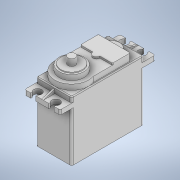
# Autodesk Inventor part: HS-485HB
Saved by Autodesk Inventor 2020 (Build 240168000, 168)
## iProperties
Created: 2023-02-03
Part Number: HS-485HB
Material: Generic
Document SubType Name: Modeling
Designer: legoo
Density: 1 g/cm^3
Appearance: Default
Author: legoo
Autodesk Inventor part; units mm, degrees
ref_plane "YZ Plane" through (0, 0, 0) normal (1, 0, 0) x (0, 1, 0)
ref_plane "XZ Plane" through (0, 0, 0) normal (0, 1, 0) x (-1, 0, 0)
sketch "Sketch1" plane through (0, 0, 0) normal (0, 1, 0) x (-1, 0, 0)
  line L0 (0, 0) -> (19.8, 0)
  line L1 (19.8, 0) -> (19.8, -40.2)
  line L2 (19.8, -40.2) -> (0, -40.2)
  line L3 (0, -40.2) -> (0, 0)
  dimension "d0" = 40.2
  dimension "d1" = 19.8
  constraints: 8 end point, 2 parallel, 1 horizontal, 1 perpendicular
  measures "d0" distance of L2.end L0.start
  measures "d1" distance of L0.start L0.end
extrude "Extrusion1" add sketch "Sketch1" along normal blind 27.7
sketch "Sketch2" plane through (0, 27.7, 0) normal (0, 1, 0) x (1, 0, 0)
  line L0 (-19.8, -6.4) -> (0, -6.4)
  line L1 (0, -6.4) -> (0, 46.6)
  line L2 (0, 46.6) -> (-19.8, 46.6)
  line L3 (-19.8, 46.6) -> (-19.8, -6.4)
  line L4 (-19.8, 40.2) -> (-19.8, 0) projected
  line L5 (0, 0) -> (0, 40.2) projected
  line L6 (-19.8, 0) -> (0, 0) projected
  dimension "d4" = 0
  dimension "d5" = 0
  dimension "d6" = 53
  dimension "d7" = 6.4
  constraints: 8 end point, 2 parallel, 1 horizontal, 1 perpendicular
  measures "d4" distance between parallel lines of L3 L4
  measures "d5" distance between parallel lines of L1 L5
  measures "d6" distance between parallel lines of L0 L2
  measures "d7" distance between parallel lines of L0 L6
extrude "Extrusion2" add sketch "Sketch2" along normal blind 2.6
sketch "Sketch3" plane through (0, 30.3, 0) normal (0, 1, 0) x (1, 0, 0)
  arc A0 (-13.5375, -5.6705) -> (-16.4375, -5.6705) centre (-14.9875, -3.95) ccw
  arc A1 (-3.4, -5.6705) -> (-6.3, -5.6705) centre (-4.85, -3.95) ccw
  arc A2 (-16.4, 45.8705) -> (-13.5, 45.8705) centre (-14.95, 44.15) ccw
  arc A3 (-6.3, 45.8705) -> (-3.4, 45.8705) centre (-4.85, 44.15) ccw
  line L0 (0, -6.4) -> (0, 46.6) projected
  line L1 (0, 46.6) -> (-19.8, 46.6) projected
  line L2 (-16.4375, -5.6705) -> (-16.4375, -6.4)
  line L3 (-13.5375, -5.6705) -> (-13.5375, -6.4)
  line L4 (-19.8, -6.4) -> (0, -6.4) projected
  line L5 (-16.4375, -6.4) -> (-13.5375, -6.4)
  line L6 (-6.3, -5.6705) -> (-6.3, -6.4)
  line L7 (-3.4, -5.6705) -> (-3.4, -6.4)
  line L8 (-6.3, -6.4) -> (-3.4, -6.4)
  line L9 (-16.4, 46.6) -> (-16.4, 45.8705)
  line L10 (-13.5, 45.8705) -> (-13.5, 46.6)
  line L11 (-6.3, 45.8705) -> (-6.3, 46.6)
  line L12 (-3.4, 45.8705) -> (-3.4, 46.6)
  line L13 (-16.4, 46.6) -> (-13.5, 46.6)
  line L14 (-6.3, 46.6) -> (-3.4, 46.6)
  point P0 (0, 0)
  dimension "d10" = 4.5
  dimension "d11" = 48.1
  dimension "d12" = 48.1
  dimension "d13" = 10.1
  dimension "d14" = 4.85
  dimension "d15" = 4.85
  dimension "d16" = 2.45
  dimension "d17" = 2.45
  dimension "d18" = 2.9
  dimension "d19" = 1.45
  dimension "d20" = 2.9
  dimension "d21" = 1.45
  dimension "d22" = 2.9
  dimension "d23" = 2.9
  dimension "d24" = 1.45
  dimension "d25" = 1.45
  constraints: 24 end point, 8 point on circle, 8 point on line, 7 vertical, 4 centre point, 3 equal radius, 1 perpendicular
  measures "d10" diameter of A0
  measures "d11" distance of A3.centre A1.centre
  measures "d12" distance of A0.centre A2.centre
  measures "d13" distance of A3.centre A2.centre
  measures "d14" distance from line of L0 A1.centre
  measures "d15" distance from line of L0 A3.centre
  measures "d16" distance from line of L1 A2.centre
  measures "d17" distance from line of L1 A3.centre
  measures "d18" distance between parallel lines of L3 L2
  measures "d19" distance from line of A0.centre L2
  measures "d20" distance between parallel lines of L7 L6
  measures "d21" distance from line of A1.centre L6
  measures "d22" distance between parallel lines of L10 L9
  measures "d23" distance between parallel lines of L12 L11
  measures "d24" distance from line of A3.centre L11
  measures "d25" distance from line of A2.centre L9
extrude "Extrusion3" cut sketch "Sketch3" against normal blind 2.6
sketch "Sketch4" plane through (0, 30.3, 0) normal (0, 1, 0) x (1, 0, 0)
  line L0 (0, 0) -> (0, 40.2) projected
  line L1 (-19.8, 0) -> (0, 0) projected
  line L2 (-19.8, 40.2) -> (-19.8, 0) projected
  line L3 (0, 40.2) -> (-19.8, 40.2) projected
extrude "Extrusion4" add sketch "Sketch4" along normal blind 3
ref_plane "Work Plane1" through (-9.4, 0, 0) normal (1, 0, 0) x (0, 0, -1)
sketch "Sketch5" plane through (-9.4, 0, 0) normal (1, 0, 0) x (0, 0, -1)
  line L0 (-6.4, 27.7) -> (-6.4, 30.3) projected
  line L1 (-6.4, 30.3) -> (0, 32.3)
  line L2 (0, 30.3) -> (-6.4, 30.3) projected
  line L3 (0, 32.3) -> (0, 30.3)
  line L4 (0, 30.3) -> (-6.4, 30.3)
  line L5 (40.2, 30.3) -> (46.6, 30.3) projected
  line L6 (40.2, 30.3) -> (46.6656, 30.3)
  line L7 (46.6656, 30.3) -> (40.2, 32.3)
  line L8 (40.2, 30.3) -> (40.2, 32.3)
  point P0 (0, 0)
  dimension "d31" = 2
  dimension "d32" = 2
  constraints: 12 end point, 3 perpendicular, 1 horizontal
  measures "d31" distance of L1.end L2.start
  measures "d32" distance of L5.start L7.end
extrude "Extrusion5" add sketch "Sketch5" against normal blind 1
sketch "Sketch6" plane through (0, 33.3, 0) normal (0, 1, 0) x (1, 0, 0)
  line L0 (0, 40.2) -> (-19.8, 40.2) projected
  line L1 (-19.8, 40.2) -> (-19.8, 0) projected
  line L2 (-19.8, 0) -> (0, 0) projected
  line L3 (0, 0) -> (0, 40.2) projected
  line L4 (-19.3, 0.5) -> (-19.3, 39.7)
  line L5 (-19.3, 39.7) -> (-0.5, 39.7)
  line L6 (-0.5, 39.7) -> (-0.5, 0.5)
  line L7 (-0.5, 0.5) -> (-19.3, 0.5)
  dimension "d35" = 0.5
  constraints: 8 end point, 3 other
  measures "d35" distance between parallel lines of L4 L1
extrude "Extrusion6" add sketch "Sketch6" along normal blind 4 contours L4 L5 L6 L7
sketch "Sketch7" plane through (0, 37.3, 0) normal (0, 1, 0) x (1, 0, 0)
  line L0 (-0.5, 39.7) -> (-19.3, 39.7) projected
  line L1 (-0.5, 0.5) -> (-0.5, 39.7) projected
  line L2 (-19.3, 39.7) -> (-0.5, 39.7)
  line L3 (-0.5, 39.7) -> (-0.5, 33.7)
  line L4 (-19.3, 33.7) -> (-19.3, 39.7)
  arc A0 (-5.3174, 33.7) -> (-14.4826, 33.7) centre (-9.9, 31.7) ccw
  line L5 (-19.3, 39.7) -> (-19.3, 0.5) projected
  line L6 (-1, 33.7) -> (-5.3174, 33.7)
  line L7 (-14.4826, 33.7) -> (-18.8, 33.7)
  line L8 (-1, 33.7) -> (-1, 23.7)
  line L9 (-1, 23.7) -> (-0.5, 23.7)
  line L10 (-0.5, 23.7) -> (-0.5, 33.7)
  line L11 (-18.8, 33.7) -> (-18.8, 23.7)
  line L12 (-18.8, 23.7) -> (-19.3, 23.7)
  line L13 (-19.3, 23.7) -> (-19.3, 33.7)
  point P0 (0, 0)
  point P1 (-0.5, 23.7)
  dimension "d39" = 10
  dimension "d40" = 9.4
  dimension "d41" = 18.8
  dimension "d61" = 0.5
  dimension "d62" = 0.5
  dimension "d63" = 10
  dimension "d64" = 10
  constraints: 22 end point, 5 parallel, 2 point on circle, 1 centre point, 1 horizontal, 1 perpendicular, 1 point on line
  measures "d39" diameter of A0
  measures "d40" distance from line of L1 A0.centre
  measures "d41" distance between parallel lines of L1 L5
  measures "d61" distance between parallel lines of L5 L11
  measures "d62" distance between parallel lines of L1 L8
  measures "d63" distance between parallel lines of L9 L6
  measures "d64" distance between parallel lines of L12 L7
extrude "Extrusion7" cut sketch "Sketch7" against normal up to surface (4 mm away)
fillet "Fillet1" radius 1 4 edges at (0, 29, 6.4) (0, 29, -46.6) (-19.8, 29, -46.6) (-19.8, 29, 6.4)
fillet "Fillet2" radius 1 8 edges at (0, 13.85, -40.2) (0, 31.8, -40.2) (0, 31.8, 0) (0, 13.85, 0) (-19.8, 13.85, -40.2) (-19.8, 31.8, -40.2) (-19.8, 13.85, 0) (-19.8, 31.8, 0)
fillet "Fillet3" radius 0.5 8 edges at (-0.2929, 33.3, -39.9071) (-9.9, 33.3, -40.2) (-19.5071, 33.3, -39.9071) (-19.8, 33.3, -20.1) (-19.5071, 33.3, -0.2929) (-9.9, 33.3, 0) (-0.2929, 33.3, -0.2929) (0, 33.3, -20.1)
sketch "Sketch8" plane through (0, 37.3, 0) normal (0, 1, 0) x (1, 0, 0)
  arc A0 (-5.3174, 33.7) -> (-14.4826, 33.7) centre (-9.9, 31.7) ccw projected
  line L0 (-14.4826, 33.7) -> (-5.3174, 33.7)
  line L1 (-19.3, 1) -> (-19.3, 23.7) projected
  arc A1 (-11.9, 23.7) -> (-7.9, 23.7) centre (-9.9, 23.7) ccw
  line L2 (-19.3, 0.5) -> (-0.5, 0.5) projected
  line L3 (-19.3, 0.5) -> (-0.5, 0.5)
  line L4 (-0.5, 0.5) -> (-0.5, 23.7)
  line L5 (-19.3, 23.7) -> (-19.3, 0.5)
  line L6 (-0.5, 23.7) -> (-7.9, 23.7)
  line L7 (-11.9, 23.7) -> (-19.3, 23.7)
  line L8 (-0.5, 23.7) -> (-7.9, 23.7)
  line L9 (-11.9, 23.7) -> (-19.3, 23.7)
  point P0 (0, 0)
  point P1 (-19.3, 33.7)
  point P2 (-0.5, 0.5)
  dimension "d49" = 4
  constraints: 16 end point, 3 parallel, 2 horizontal, 2 point on circle, 1 centre point, 1 perpendicular
  measures "d49" diameter of A1
extrude "Extrusion8" cut sketch "Sketch8" against normal blind 1
sketch "Sketch9" plane through (0, 36.3, 0) normal (0, 1, 0) x (1, 0, 0)
  arc A0 (-18.8, 12.9249) -> (-1, 12.9249) centre (-9.9, 9.9) ccw
  line L0 (-18.8, 0) -> (-1, 0) projected
  line L1 (-18.8, 23.7) -> (-11.9, 23.7) projected
  line L2 (-18.8, 23.7) -> (-18.8, 12.9249)
  line L3 (-7.9, 23.7) -> (-1, 23.7) projected
  line L4 (-1, 23.7) -> (-1, 12.9249)
  line L5 (-18.8, 33.7) -> (-18.8, 23.7) projected
  line L6 (-19.3, 23.7) -> (-18.8, 23.7) projected
  line L7 (-18.8, 23.7) -> (-19.3, 23.7)
  line L8 (-19.3, 23.7) -> (-19.3, 0.5)
  line L9 (-0.5, 23.7) -> (-0.5, 1) projected
  line L10 (-1, 23.7) -> (-0.5, 23.7)
  line L11 (-0.5, 0.5) -> (-19.3, 0.5) projected
  line L12 (-0.5, 23.7) -> (-0.5, 0.5)
  line L13 (-0.5, 0.5) -> (-19.3, 0.5)
  point P0 (0, 0)
  point P1 (-19.3, 9.9)
  point P2 (-0.5, 1)
  point P3 (-0.5, 9.9)
  point P4 (-9.9, 0.5)
  dimension "d54" = 18.8
  dimension "d56" = 9.9
  constraints: 16 end point, 4 perpendicular, 2 horizontal, 2 point on circle, 1 centre point, 1 vertical
  measures "d54" diameter of A0
  measures "d56" distance from line of L0 A0.centre
extrude "Extrusion9" cut sketch "Sketch9" against normal up to surface (3 mm away)
fillet "Fillet4" radius 0.5 4 edges at (-1, 35.3, -33.7) (-1, 36.8, -23.7) (-18.8, 36.8, -23.7) (-18.8, 35.3, -33.7)
sketch "Sketch10" plane through (0, 36.3, 0) normal (0, 1, 0) x (1, 0, 0)
  arc A0 (-18.8, 12.9249) -> (-1, 12.9249) centre (-9.9, 9.9) ccw projected
  circle A1 centre (-9.9, 9.9) radius 7
  point P0 (0, 0)
  dimension "d66" = 14
  constraints: 1 centre point, 1 coincident
  measures "d66" diameter of A1
extrude "Extrusion10" add sketch "Sketch10" along normal blind 3.4
sketch "Sketch11" plane through (-9.9, 39.7, -9.9) normal (0, 1, 0) x (1, 0, 0)
  circle A0 centre (0, 0) radius 7 projected
  circle A1 centre (0, 0) radius 6
  point P0 (9.9, -9.9)
  dimension "d69" = 1
  constraints: 1 centre point
  measures "d69" radial gap between concentric circles of A0 A1
extrude "Extrusion11" cut sketch "Sketch11" against normal blind 0.5
sketch "Sketch12" plane through (-9.9, 39.7, -9.9) normal (0, 1, 0) x (1, 0, 0)
  circle A0 centre (0, 0) radius 6 projected
  circle A1 centre (0, 0) radius 2.1
  point P0 (9.9, -9.9)
  dimension "d72" = 4.2
  constraints: 1 centre point, 1 coincident
  measures "d72" diameter of A1
extrude "Extrusion12" add sketch "Sketch12" along normal blind 3.7 contours A1
equation "\"d40\" = 0.5 * d41"
body "Solid1"
